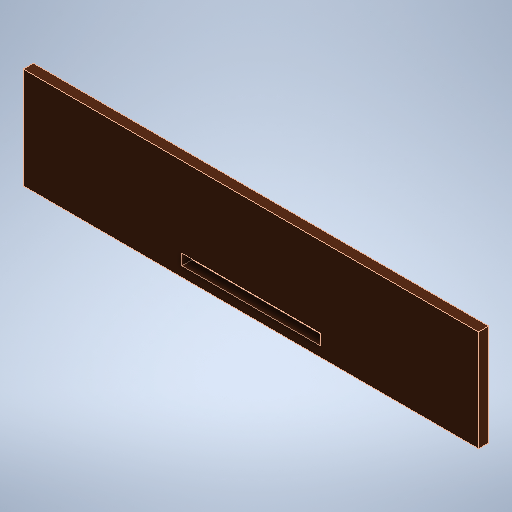
# Autodesk Inventor part: Path Side Wall
Saved by Autodesk Inventor 2025.4 (Build 294407000, 407)
## iProperties
Created: 2026-04-06
Part Number: Path Side Wall
Material: Generic
Document SubType Name: Sheet Metal
Designer: lenovo
Density: 1 g/cm^3
Sheet Metal Rule: Default_mm
Appearance: Default(1)
Author: lenovo
Autodesk Inventor part; units mm, degrees
ref_plane "YZ Plane" through (0, 0, 0) normal (1, 0, 0) x (0, 1, 0)
ref_plane "XZ Plane" through (0, 0, 0) normal (0, 1, 0) x (-1, 0, 0)
ref_plane "XY Plane" through (0, 0, 0) normal (0, 0, 1) x (1, 0, 0)
sketch "Sketch1" plane through (0, 0, 0) normal (0, 0, 1) x (1, 0, 0)
  line L0 (-67.5, -15) -> (67.5, -15)
  line L1 (67.5, -15) -> (67.5, 15)
  line L2 (67.5, 15) -> (-67.5, 15)
  line L3 (-67.5, 15) -> (-67.5, -15)
  line L4 (-67.5, -15) -> (67.5, 15) construction
  line L5 (67.5, -15) -> (-67.5, 15) construction
  line L6 (-20.5, -8.8) -> (20.5, -8.8)
  line L7 (20.5, -8.8) -> (20.5, -12)
  line L8 (20.5, -12) -> (-20.5, -12)
  line L9 (-20.5, -12) -> (-20.5, -8.8)
  line L10 (-20.5, -8.8) -> (20.5, -12) construction
  line L11 (20.5, -8.8) -> (-20.5, -12) construction
  point P0 (0, 0)
  point P1 (0, -10.4)
  point P2 (0, -8.8)
  dimension "d0" = 135
  dimension "d1" = 30
  dimension "d5" = 41
  dimension "d6" = 3
  dimension "d7" = 3.2
  measures "d0" distance of L1.end L2.end
  measures "d1" distance of L2.end L0.start
  measures "d5" distance of L6.start L6.end
  measures "d6" distance between parallel lines of L0 L8
  measures "d7" distance of L8.end L6.start
extrude "Plate1" add sketch "Sketch1" along normal mid plane 3
equation "\"d4\" = Thickness"
equation "\"BendRadius\" = Thickness"
equation "\"BendReliefWidth\" = Thickness"
equation "\"BendReliefDepth\" = 0.5 * Thickness"
equation "\"CornerReliefSize\" = 4 * Thickness"
equation "\"MinimumRemnant\" = 2 * Thickness"
equation "\"TransitionRadius\" = BendRadius"
equation "\"JacobiRadiusSize\" = BendRadius"
equation "\"GapSize\" = Thickness"
equation "\"Thickness\" = 3"
body "Solid1"
